Autodesk Fusion 360 part; units mm, degrees
(part 12 of 40)
  spline S70 degree 5 poles (151.3635, 144.3049) (151.3327, 144.3021) (151.2711, 144.2971) (151.1787, 144.2922) (151.0554, 144.2903) (150.901, 144.2944) (150.7464, 144.3031) (150.5917, 144.3146) (150.437, 144.3277) (150.2822, 144.3417) (150.1275, 144.3569) (149.9727, 144.3735) (149.818, 144.392) (149.6632, 144.4129) (149.5085, 144.4359) (149.3538, 144.461) (149.1991, 144.4879) (149.0445, 144.5162) (148.8899, 144.5458) (148.7354, 144.5767) (148.5809, 144.6087) (148.4265, 144.6421) (148.2722, 144.6768) (148.118, 144.7129) (147.9638, 144.7503) (147.8098, 144.7891) (147.6558, 144.8291) (147.5019, 144.8703) (147.3481, 144.9127) (147.1944, 144.9561) (147.0408, 145.0007) (146.8873, 145.0464) (146.734, 145.0932) (146.5807, 145.1411) (146.4276, 145.1901) (146.2746, 145.2401) (146.1217, 145.2913) (145.9689, 145.3434) (145.8162, 145.3965) (145.6637, 145.4507) (145.5114, 145.5058) (145.3591, 145.562) (145.207, 145.619) (145.055, 145.6771) (144.9032, 145.7361) (144.7516, 145.7961) (144.6, 145.857) (144.4487, 145.9188) (144.2975, 145.9815) (144.1464, 146.0452) (143.9955, 146.1097) (143.8448, 146.1751) (143.6942, 146.2415) (143.5438, 146.3087) (143.3936, 146.3767) (143.2435, 146.4457) (143.0936, 146.5154) (142.9439, 146.5861) (142.7944, 146.6575) (142.645, 146.7299) (142.4958, 146.803) (142.3468, 146.877) (142.198, 146.9518) (142.0494, 147.0274) (141.9009, 147.1038) (141.7527, 147.181) (141.6046, 147.259) (141.4568, 147.3378) (141.3091, 147.4174) (141.1617, 147.4977) (141.0144, 147.5789) (140.8968, 147.6444) (140.8086, 147.6939) (140.7499, 147.7271) (140.7205, 147.7437) knots 0 0 0 0 0 0 0.01428571 0.02857143 0.04285714 0.05714286 0.07142857 0.08571429 0.1 0.11428571 0.12857143 0.14285714 0.15714286 0.17142857 0.18571429 0.2 0.21428571 0.22857143 0.24285714 0.25714286 0.27142857 0.28571429 0.3 0.31428571 0.32857143 0.34285714 0.35714286 0.37142857 0.38571429 0.4 0.41428571 0.42857143 0.44285714 0.45714286 0.47142857 0.48571429 0.5 0.51428571 0.52857143 0.54285714 0.55714286 0.57142857 0.58571429 0.6 0.61428571 0.62857143 0.64285714 0.65714286 0.67142857 0.68571429 0.7 0.71428571 0.72857143 0.74285714 0.75714286 0.77142857 0.78571429 0.8 0.81428571 0.82857143 0.84285714 0.85714286 0.87142857 0.88571429 0.9 0.91428571 0.92857143 0.94285714 0.95714286 0.97142857 0.98571429 1 1 1 1 1 1
  line L5257 (151.3635, 144.3049) -> (151.3327, 144.3021) construction
  line L5258 (151.3327, 144.3021) -> (151.2711, 144.2971) construction
  line L5259 (151.2711, 144.2971) -> (151.1787, 144.2922) construction
  line L5260 (151.1787, 144.2922) -> (151.0554, 144.2903) construction
  line L5261 (151.0554, 144.2903) -> (150.901, 144.2944) construction
  line L5262 (150.901, 144.2944) -> (150.7464, 144.3031) construction
  line L5263 (150.7464, 144.3031) -> (150.5917, 144.3146) construction
  line L5264 (150.5917, 144.3146) -> (150.437, 144.3277) construction
  line L5265 (150.437, 144.3277) -> (150.2822, 144.3417) construction
  line L5266 (150.2822, 144.3417) -> (150.1275, 144.3569) construction
  line L5267 (150.1275, 144.3569) -> (149.9727, 144.3735) construction
  line L5268 (149.9727, 144.3735) -> (149.818, 144.392) construction
  line L5269 (149.818, 144.392) -> (149.6632, 144.4129) construction
  line L5270 (149.6632, 144.4129) -> (149.5085, 144.4359) construction
  line L5271 (149.5085, 144.4359) -> (149.3538, 144.461) construction
  line L5272 (149.3538, 144.461) -> (149.1991, 144.4879) construction
  line L5273 (149.1991, 144.4879) -> (149.0445, 144.5162) construction
  line L5274 (149.0445, 144.5162) -> (148.8899, 144.5458) construction
  line L5275 (148.8899, 144.5458) -> (148.7354, 144.5767) construction
  line L5276 (148.7354, 144.5767) -> (148.5809, 144.6087) construction
  line L5277 (148.5809, 144.6087) -> (148.4265, 144.6421) construction
  line L5278 (148.4265, 144.6421) -> (148.2722, 144.6768) construction
  line L5279 (148.2722, 144.6768) -> (148.118, 144.7129) construction
  line L5280 (148.118, 144.7129) -> (147.9638, 144.7503) construction
  line L5281 (147.9638, 144.7503) -> (147.8098, 144.7891) construction
  line L5282 (147.8098, 144.7891) -> (147.6558, 144.8291) construction
  line L5283 (147.6558, 144.8291) -> (147.5019, 144.8703) construction
  line L5284 (147.5019, 144.8703) -> (147.3481, 144.9127) construction
  line L5285 (147.3481, 144.9127) -> (147.1944, 144.9561) construction
  line L5286 (147.1944, 144.9561) -> (147.0408, 145.0007) construction
  line L5287 (147.0408, 145.0007) -> (146.8873, 145.0464) construction
  line L5288 (146.8873, 145.0464) -> (146.734, 145.0932) construction
  line L5289 (146.734, 145.0932) -> (146.5807, 145.1411) construction
  line L5290 (146.5807, 145.1411) -> (146.4276, 145.1901) construction
  line L5291 (146.4276, 145.1901) -> (146.2746, 145.2401) construction
  line L5292 (146.2746, 145.2401) -> (146.1217, 145.2913) construction
  line L5293 (146.1217, 145.2913) -> (145.9689, 145.3434) construction
  line L5294 (145.9689, 145.3434) -> (145.8162, 145.3965) construction
  line L5295 (145.8162, 145.3965) -> (145.6637, 145.4507) construction
  line L5296 (145.6637, 145.4507) -> (145.5114, 145.5058) construction
  line L5297 (145.5114, 145.5058) -> (145.3591, 145.562) construction
  line L5298 (145.3591, 145.562) -> (145.207, 145.619) construction
  line L5299 (145.207, 145.619) -> (145.055, 145.6771) construction
  line L5300 (145.055, 145.6771) -> (144.9032, 145.7361) construction
  line L5301 (144.9032, 145.7361) -> (144.7516, 145.7961) construction
  line L5302 (144.7516, 145.7961) -> (144.6, 145.857) construction
  line L5303 (144.6, 145.857) -> (144.4487, 145.9188) construction
  line L5304 (144.4487, 145.9188) -> (144.2975, 145.9815) construction
  line L5305 (144.2975, 145.9815) -> (144.1464, 146.0452) construction
  line L5306 (144.1464, 146.0452) -> (143.9955, 146.1097) construction
  line L5307 (143.9955, 146.1097) -> (143.8448, 146.1751) construction
  line L5308 (143.8448, 146.1751) -> (143.6942, 146.2415) construction
  line L5309 (143.6942, 146.2415) -> (143.5438, 146.3087) construction
  line L5310 (143.5438, 146.3087) -> (143.3936, 146.3767) construction
  line L5311 (143.3936, 146.3767) -> (143.2435, 146.4457) construction
  line L5312 (143.2435, 146.4457) -> (143.0936, 146.5154) construction
  line L5313 (143.0936, 146.5154) -> (142.9439, 146.5861) construction
  line L5314 (142.9439, 146.5861) -> (142.7944, 146.6575) construction
  line L5315 (142.7944, 146.6575) -> (142.645, 146.7299) construction
  line L5316 (142.645, 146.7299) -> (142.4958, 146.803) construction
  line L5317 (142.4958, 146.803) -> (142.3468, 146.877) construction
  line L5318 (142.3468, 146.877) -> (142.198, 146.9518) construction
  line L5319 (142.198, 146.9518) -> (142.0494, 147.0274) construction
  line L5320 (142.0494, 147.0274) -> (141.9009, 147.1038) construction
  line L5321 (141.9009, 147.1038) -> (141.7527, 147.181) construction
  line L5322 (141.7527, 147.181) -> (141.6046, 147.259) construction
  line L5323 (141.6046, 147.259) -> (141.4568, 147.3378) construction
  line L5324 (141.4568, 147.3378) -> (141.3091, 147.4174) construction
  line L5325 (141.3091, 147.4174) -> (141.1617, 147.4977) construction
  line L5326 (141.1617, 147.4977) -> (141.0144, 147.5789) construction
  line L5327 (141.0144, 147.5789) -> (140.8968, 147.6444) construction
  line L5328 (140.8968, 147.6444) -> (140.8086, 147.6939) construction
  line L5329 (140.8086, 147.6939) -> (140.7499, 147.7271) construction
  line L5330 (140.7499, 147.7271) -> (140.7205, 147.7437) construction
  arc A144 (140.7205, 152.2563) -> (140.7205, 147.7437) centre (212.132, 150) ccw
  spline S71 degree 5 poles (159.6217, 118.8885) (159.5952, 118.8728) (159.5425, 118.8406) (159.4648, 118.7903) (159.3639, 118.7193) (159.2414, 118.6252) (159.1214, 118.5273) (159.0031, 118.4271) (158.8856, 118.3256) (158.7686, 118.2233) (158.6523, 118.12) (158.5369, 118.0156) (158.4226, 117.9097) (158.3096, 117.8019) (158.198, 117.6923) (158.0876, 117.581) (157.9783, 117.4684) (157.8698, 117.3545) (157.7622, 117.2397) (157.6553, 117.124) (157.5492, 117.0073) (157.4439, 116.8895) (157.3394, 116.7708) (157.2359, 116.6509) (157.1332, 116.53) (157.0313, 116.4081) (156.9303, 116.2852) (156.83, 116.1614) (156.7305, 116.0367) (156.6317, 115.9112) (156.5336, 115.7849) (156.4363, 115.6577) (156.3397, 115.5297) (156.2439, 115.4009) (156.1488, 115.2712) (156.0544, 115.1408) (155.9608, 115.0095) (155.8678, 114.8776) (155.7756, 114.7448) (155.684, 114.6114) (155.5932, 114.4772) (155.503, 114.3423) (155.4135, 114.2067) (155.3247, 114.0705) (155.2365, 113.9335) (155.1491, 113.7958) (155.0623, 113.6575) (154.9762, 113.5185) (154.8907, 113.3789) (154.8059, 113.2386) (154.7218, 113.0977) (154.6383, 112.9562) (154.5555, 112.814) (154.4733, 112.6712) (154.3917, 112.5279) (154.3108, 112.3839) (154.2306, 112.2393) (154.151, 112.0942) (154.072, 111.9485) (153.9937, 111.8022) (153.916, 111.6553) (153.8389, 111.5079) (153.7625, 111.3599) (153.6867, 111.2114) (153.6115, 111.0623) (153.537, 110.9127) (153.463, 110.7626) (153.3897, 110.6119) (153.3171, 110.4607) (153.245, 110.3091) (153.1736, 110.1569) (153.1169, 110.0347) (153.0747, 109.9428) (153.0467, 109.8815) (153.0327, 109.8508) knots 0 0 0 0 0 0 0.01428571 0.02857143 0.04285714 0.05714286 0.07142857 0.08571429 0.1 0.11428571 0.12857143 0.14285714 0.15714286 0.17142857 0.18571429 0.2 0.21428571 0.22857143 0.24285714 0.25714286 0.27142857 0.28571429 0.3 0.31428571 0.32857143 0.34285714 0.35714286 0.37142857 0.38571429 0.4 0.41428571 0.42857143 0.44285714 0.45714286 0.47142857 0.48571429 0.5 0.51428571 0.52857143 0.54285714 0.55714286 0.57142857 0.58571429 0.6 0.61428571 0.62857143 0.64285714 0.65714286 0.67142857 0.68571429 0.7 0.71428571 0.72857143 0.74285714 0.75714286 0.77142857 0.78571429 0.8 0.81428571 0.82857143 0.84285714 0.85714286 0.87142857 0.88571429 0.9 0.91428571 0.92857143 0.94285714 0.95714286 0.97142857 0.98571429 1 1 1 1 1 1
  line L5331 (159.6217, 118.8885) -> (159.5952, 118.8728) construction
  line L5332 (159.5952, 118.8728) -> (159.5425, 118.8406) construction
  line L5333 (159.5425, 118.8406) -> (159.4648, 118.7903) construction
  line L5334 (159.4648, 118.7903) -> (159.3639, 118.7193) construction
  line L5335 (159.3639, 118.7193) -> (159.2414, 118.6252) construction
  line L5336 (159.2414, 118.6252) -> (159.1214, 118.5273) construction
  line L5337 (159.1214, 118.5273) -> (159.0031, 118.4271) construction
  line L5338 (159.0031, 118.4271) -> (158.8856, 118.3256) construction
  line L5339 (158.8856, 118.3256) -> (158.7686, 118.2233) construction
  line L5340 (158.7686, 118.2233) -> (158.6523, 118.12) construction
  line L5341 (158.6523, 118.12) -> (158.5369, 118.0156) construction
  line L5342 (158.5369, 118.0156) -> (158.4226, 117.9097) construction
  line L5343 (158.4226, 117.9097) -> (158.3096, 117.8019) construction
  line L5344 (158.3096, 117.8019) -> (158.198, 117.6923) construction
  line L5345 (158.198, 117.6923) -> (158.0876, 117.581) construction
  line L5346 (158.0876, 117.581) -> (157.9783, 117.4684) construction
  line L5347 (157.9783, 117.4684) -> (157.8698, 117.3545) construction
  line L5348 (157.8698, 117.3545) -> (157.7622, 117.2397) construction
  line L5349 (157.7622, 117.2397) -> (157.6553, 117.124) construction
  line L5350 (157.6553, 117.124) -> (157.5492, 117.0073) construction
  line L5351 (157.5492, 117.0073) -> (157.4439, 116.8895) construction
  line L5352 (157.4439, 116.8895) -> (157.3394, 116.7708) construction
  line L5353 (157.3394, 116.7708) -> (157.2359, 116.6509) construction
  line L5354 (157.2359, 116.6509) -> (157.1332, 116.53) construction
  line L5355 (157.1332, 116.53) -> (157.0313, 116.4081) construction
  line L5356 (157.0313, 116.4081) -> (156.9303, 116.2852) construction
  line L5357 (156.9303, 116.2852) -> (156.83, 116.1614) construction
  line L5358 (156.83, 116.1614) -> (156.7305, 116.0367) construction
  line L5359 (156.7305, 116.0367) -> (156.6317, 115.9112) construction
  line L5360 (156.6317, 115.9112) -> (156.5336, 115.7849) construction
  line L5361 (156.5336, 115.7849) -> (156.4363, 115.6577) construction
  line L5362 (156.4363, 115.6577) -> (156.3397, 115.5297) construction
  line L5363 (156.3397, 115.5297) -> (156.2439, 115.4009) construction
  line L5364 (156.2439, 115.4009) -> (156.1488, 115.2712) construction
  line L5365 (156.1488, 115.2712) -> (156.0544, 115.1408) construction
  line L5366 (156.0544, 115.1408) -> (155.9608, 115.0095) construction
  line L5367 (155.9608, 115.0095) -> (155.8678, 114.8776) construction
  line L5368 (155.8678, 114.8776) -> (155.7756, 114.7448) construction
  line L5369 (155.7756, 114.7448) -> (155.684, 114.6114) construction
  line L5370 (155.684, 114.6114) -> (155.5932, 114.4772) construction
  line L5371 (155.5932, 114.4772) -> (155.503, 114.3423) construction
  line L5372 (155.503, 114.3423) -> (155.4135, 114.2067) construction
  line L5373 (155.4135, 114.2067) -> (155.3247, 114.0705) construction
  line L5374 (155.3247, 114.0705) -> (155.2365, 113.9335) construction
  line L5375 (155.2365, 113.9335) -> (155.1491, 113.7958) construction
  line L5376 (155.1491, 113.7958) -> (155.0623, 113.6575) construction
  line L5377 (155.0623, 113.6575) -> (154.9762, 113.5185) construction
  line L5378 (154.9762, 113.5185) -> (154.8907, 113.3789) construction
  line L5379 (154.8907, 113.3789) -> (154.8059, 113.2386) construction
  line L5380 (154.8059, 113.2386) -> (154.7218, 113.0977) construction
  line L5381 (154.7218, 113.0977) -> (154.6383, 112.9562) construction
  line L5382 (154.6383, 112.9562) -> (154.5555, 112.814) construction
  line L5383 (154.5555, 112.814) -> (154.4733, 112.6712) construction
  line L5384 (154.4733, 112.6712) -> (154.3917, 112.5279) construction
  line L5385 (154.3917, 112.5279) -> (154.3108, 112.3839) construction
  line L5386 (154.3108, 112.3839) -> (154.2306, 112.2393) construction
  line L5387 (154.2306, 112.2393) -> (154.151, 112.0942) construction
  line L5388 (154.151, 112.0942) -> (154.072, 111.9485) construction
  line L5389 (154.072, 111.9485) -> (153.9937, 111.8022) construction
  line L5390 (153.9937, 111.8022) -> (153.916, 111.6553) construction
  line L5391 (153.916, 111.6553) -> (153.8389, 111.5079) construction
  line L5392 (153.8389, 111.5079) -> (153.7625, 111.3599) construction
  line L5393 (153.7625, 111.3599) -> (153.6867, 111.2114) construction
  line L5394 (153.6867, 111.2114) -> (153.6115, 111.0623) construction
  line L5395 (153.6115, 111.0623) -> (153.537, 110.9127) construction
  line L5396 (153.537, 110.9127) -> (153.463, 110.7626) construction
  line L5397 (153.463, 110.7626) -> (153.3897, 110.6119) construction
  line L5398 (153.3897, 110.6119) -> (153.3171, 110.4607) construction
  line L5399 (153.3171, 110.4607) -> (153.245, 110.3091) construction
  line L5400 (153.245, 110.3091) -> (153.1736, 110.1569) construction
  line L5401 (153.1736, 110.1569) -> (153.1169, 110.0347) construction
  line L5402 (153.1169, 110.0347) -> (153.0747, 109.9428) construction
  line L5403 (153.0747, 109.9428) -> (153.0467, 109.8815) construction
  line L5404 (153.0467, 109.8815) -> (153.0327, 109.8508) construction
  arc A145 (152.9878, 155.5428) -> (155.1583, 157.2806) centre (153.1745, 157.5341) ccw
  arc A146 (160.1966, 125.4699) -> (157.5954, 126.4519) centre (158.3882, 124.6158) ccw
  arc A147 (155.6851, 193.8) -> (153.0327, 190.1492) centre (212.132, 150) ccw
  spline S72 degree 5 poles (152.5778, 136.6378) (152.5477, 136.631) (152.4876, 136.6167) (152.3982, 136.5929) (152.2803, 136.5565) (152.1347, 136.5049) (151.9904, 136.4489) (151.8468, 136.3901) (151.7037, 136.3299) (151.5609, 136.2687) (151.4184, 136.2065) (151.2763, 136.1429) (151.1349, 136.0774) (150.9941, 136.0098) (150.8541, 135.94) (150.7147, 135.8684) (150.5759, 135.795) (150.4376, 135.7203) (150.2998, 135.6443) (150.1623, 135.5673) (150.0253, 135.4891) (149.8888, 135.4096) (149.7528, 135.3289) (149.6172, 135.247) (149.4822, 135.1637) (149.3477, 135.0792) (149.2136, 134.9936) (149.08, 134.9068) (148.9468, 134.819) (148.814, 134.7302) (148.6817, 134.6403) (148.5499, 134.5494) (148.4185, 134.4575) (148.2875, 134.3646) (148.157, 134.2707) (148.027, 134.1758) (147.8974, 134.08) (147.7682, 133.9832) (147.6394, 133.8854) (147.5111, 133.7868) (147.3832, 133.6873) (147.2558, 133.5869) (147.1288, 133.4856) (147.0022, 133.3834) (146.876, 133.2804) (146.7503, 133.1765) (146.625, 133.0717) (146.5002, 132.9662) (146.3758, 132.8598) (146.2518, 132.7526) (146.1282, 132.6445) (146.0051, 132.5357) (145.8823, 132.4261) (145.7601, 132.3158) (145.6382, 132.2046) (145.5168, 132.0927) (145.3958, 131.98) (145.2752, 131.8665) (145.1551, 131.7523) (145.0354, 131.6374) (144.9161, 131.5218) (144.7973, 131.4054) (144.6789, 131.2882) (144.5609, 131.1704) (144.4433, 131.0519) (144.3262, 130.9326) (144.2095, 130.8127) (144.0932, 130.6921) (143.9774, 130.5707) (143.862, 130.4488) (143.747, 130.3261) (143.6553, 130.2274) (143.5868, 130.1531) (143.5412, 130.1034) (143.5184, 130.0785) knots 0 0 0 0 0 0 0.01428571 0.02857143 0.04285714 0.05714286 0.07142857 0.08571429 0.1 0.11428571 0.12857143 0.14285714 0.15714286 0.17142857 0.18571429 0.2 0.21428571 0.22857143 0.24285714 0.25714286 0.27142857 0.28571429 0.3 0.31428571 0.32857143 0.34285714 0.35714286 0.37142857 0.38571429 0.4 0.41428571 0.42857143 0.44285714 0.45714286 0.47142857 0.48571429 0.5 0.51428571 0.52857143 0.54285714 0.55714286 0.57142857 0.58571429 0.6 0.61428571 0.62857143 0.64285714 0.65714286 0.67142857 0.68571429 0.7 0.71428571 0.72857143 0.74285714 0.75714286 0.77142857 0.78571429 0.8 0.81428571 0.82857143 0.84285714 0.85714286 0.87142857 0.88571429 0.9 0.91428571 0.92857143 0.94285714 0.95714286 0.97142857 0.98571429 1 1 1 1 1 1
  line L5405 (152.5778, 136.6378) -> (152.5477, 136.631) construction
  line L5406 (152.5477, 136.631) -> (152.4876, 136.6167) construction
  line L5407 (152.4876, 136.6167) -> (152.3982, 136.5929) construction
  line L5408 (152.3982, 136.5929) -> (152.2803, 136.5565) construction
  line L5409 (152.2803, 136.5565) -> (152.1347, 136.5049) construction
  line L5410 (152.1347, 136.5049) -> (151.9904, 136.4489) construction
  line L5411 (151.9904, 136.4489) -> (151.8468, 136.3901) construction
  line L5412 (151.8468, 136.3901) -> (151.7037, 136.3299) construction
  line L5413 (151.7037, 136.3299) -> (151.5609, 136.2687) construction
  line L5414 (151.5609, 136.2687) -> (151.4184, 136.2065) construction
  line L5415 (151.4184, 136.2065) -> (151.2763, 136.1429) construction
  line L5416 (151.2763, 136.1429) -> (151.1349, 136.0774) construction
  line L5417 (151.1349, 136.0774) -> (150.9941, 136.0098) construction
  line L5418 (150.9941, 136.0098) -> (150.8541, 135.94) construction
  line L5419 (150.8541, 135.94) -> (150.7147, 135.8684) construction
  line L5420 (150.7147, 135.8684) -> (150.5759, 135.795) construction
  line L5421 (150.5759, 135.795) -> (150.4376, 135.7203) construction
  line L5422 (150.4376, 135.7203) -> (150.2998, 135.6443) construction
  line L5423 (150.2998, 135.6443) -> (150.1623, 135.5673) construction
  line L5424 (150.1623, 135.5673) -> (150.0253, 135.4891) construction
  line L5425 (150.0253, 135.4891) -> (149.8888, 135.4096) construction
  line L5426 (149.8888, 135.4096) -> (149.7528, 135.3289) construction
  line L5427 (149.7528, 135.3289) -> (149.6172, 135.247) construction
  line L5428 (149.6172, 135.247) -> (149.4822, 135.1637) construction
  line L5429 (149.4822, 135.1637) -> (149.3477, 135.0792) construction
  line L5430 (149.3477, 135.0792) -> (149.2136, 134.9936) construction
  line L5431 (149.2136, 134.9936) -> (149.08, 134.9068) construction
  line L5432 (149.08, 134.9068) -> (148.9468, 134.819) construction
  line L5433 (148.9468, 134.819) -> (148.814, 134.7302) construction
  line L5434 (148.814, 134.7302) -> (148.6817, 134.6403) construction
  line L5435 (148.6817, 134.6403) -> (148.5499, 134.5494) construction
  line L5436 (148.5499, 134.5494) -> (148.4185, 134.4575) construction
  line L5437 (148.4185, 134.4575) -> (148.2875, 134.3646) construction
  line L5438 (148.2875, 134.3646) -> (148.157, 134.2707) construction
  line L5439 (148.157, 134.2707) -> (148.027, 134.1758) construction
  line L5440 (148.027, 134.1758) -> (147.8974, 134.08) construction
  line L5441 (147.8974, 134.08) -> (147.7682, 133.9832) construction
  line L5442 (147.7682, 133.9832) -> (147.6394, 133.8854) construction
  line L5443 (147.6394, 133.8854) -> (147.5111, 133.7868) construction
  line L5444 (147.5111, 133.7868) -> (147.3832, 133.6873) construction
  line L5445 (147.3832, 133.6873) -> (147.2558, 133.5869) construction
  line L5446 (147.2558, 133.5869) -> (147.1288, 133.4856) construction
  line L5447 (147.1288, 133.4856) -> (147.0022, 133.3834) construction
  line L5448 (147.0022, 133.3834) -> (146.876, 133.2804) construction
  line L5449 (146.876, 133.2804) -> (146.7503, 133.1765) construction
  line L5450 (146.7503, 133.1765) -> (146.625, 133.0717) construction
  line L5451 (146.625, 133.0717) -> (146.5002, 132.9662) construction
  line L5452 (146.5002, 132.9662) -> (146.3758, 132.8598) construction
  line L5453 (146.3758, 132.8598) -> (146.2518, 132.7526) construction
  line L5454 (146.2518, 132.7526) -> (146.1282, 132.6445) construction
  line L5455 (146.1282, 132.6445) -> (146.0051, 132.5357) construction
  line L5456 (146.0051, 132.5357) -> (145.8823, 132.4261) construction
  line L5457 (145.8823, 132.4261) -> (145.7601, 132.3158) construction
  line L5458 (145.7601, 132.3158) -> (145.6382, 132.2046) construction
  line L5459 (145.6382, 132.2046) -> (145.5168, 132.0927) construction
  line L5460 (145.5168, 132.0927) -> (145.3958, 131.98) construction
  line L5461 (145.3958, 131.98) -> (145.2752, 131.8665) construction
  line L5462 (145.2752, 131.8665) -> (145.1551, 131.7523) construction
  line L5463 (145.1551, 131.7523) -> (145.0354, 131.6374) construction
  line L5464 (145.0354, 131.6374) -> (144.9161, 131.5218) construction
  line L5465 (144.9161, 131.5218) -> (144.7973, 131.4054) construction
  line L5466 (144.7973, 131.4054) -> (144.6789, 131.2882) construction
  line L5467 (144.6789, 131.2882) -> (144.5609, 131.1704) construction
  line L5468 (144.5609, 131.1704) -> (144.4433, 131.0519) construction
  line L5469 (144.4433, 131.0519) -> (144.3262, 130.9326) construction
  line L5470 (144.3262, 130.9326) -> (144.2095, 130.8127) construction
  line L5471 (144.2095, 130.8127) -> (144.0932, 130.6921) construction
  line L5472 (144.0932, 130.6921) -> (143.9774, 130.5707) construction
  line L5473 (143.9774, 130.5707) -> (143.862, 130.4488) construction
  line L5474 (143.862, 130.4488) -> (143.747, 130.3261) construction
  line L5475 (143.747, 130.3261) -> (143.6553, 130.2274) construction
  line L5476 (143.6553, 130.2274) -> (143.5868, 130.1531) construction
  line L5477 (143.5868, 130.1531) -> (143.5412, 130.1034) construction
  line L5478 (143.5412, 130.1034) -> (143.5184, 130.0785) construction
  spline S73 degree 5 poles (151.3635, 155.6951) (151.3327, 155.6979) (151.2711, 155.7029) (151.1787, 155.7078) (151.0554, 155.7097) (150.901, 155.7056) (150.7464, 155.6969) (150.5917, 155.6854) (150.437, 155.6723) (150.2822, 155.6583) (150.1275, 155.6431) (149.9727, 155.6265) (149.818, 155.608) (149.6632, 155.5871) (149.5085, 155.5641) (149.3538, 155.539) (149.1991, 155.5121) (149.0445, 155.4838) (148.8899, 155.4542) (148.7354, 155.4233) (148.5809, 155.3913) (148.4265, 155.3579) (148.2722, 155.3232) (148.118, 155.2871) (147.9638, 155.2497) (147.8098, 155.2109) (147.6558, 155.1709) (147.5019, 155.1297) (147.3481, 155.0873) (147.1944, 155.0439) (147.0408, 154.9993) (146.8873, 154.9536) (146.734, 154.9068) (146.5807, 154.8589) (146.4276, 154.8099) (146.2746, 154.7599) (146.1217, 154.7087) (145.9689, 154.6566) (145.8162, 154.6035) (145.6637, 154.5493) (145.5114, 154.4942) (145.3591, 154.438) (145.207, 154.381) (145.055, 154.3229) (144.9032, 154.2639) (144.7516, 154.2039) (144.6, 154.143) (144.4487, 154.0812) (144.2975, 154.0185) (144.1464, 153.9548) (143.9955, 153.8903) (143.8448, 153.8249) (143.6942, 153.7585) (143.5438, 153.6913) (143.3936, 153.6233) (143.2435, 153.5543) (143.0936, 153.4846) (142.9439, 153.4139) (142.7944, 153.3425) (142.645, 153.2701) (142.4958, 153.197) (142.3468, 153.123) (142.198, 153.0482) (142.0494, 152.9726) (141.9009, 152.8962) (141.7527, 152.819) (141.6046, 152.741) (141.4568, 152.6622) (141.3091, 152.5826) (141.1617, 152.5023) (141.0144, 152.4211) (140.8968, 152.3556) (140.8086, 152.3061) (140.7499, 152.2729) (140.7205, 152.2563) knots 0 0 0 0 0 0 0.01428571 0.02857143 0.04285714 0.05714286 0.07142857 0.08571429 0.1 0.11428571 0.12857143 0.14285714 0.15714286 0.17142857 0.18571429 0.2 0.21428571 0.22857143 0.24285714 0.25714286 0.27142857 0.28571429 0.3 0.31428571 0.32857143 0.34285714 0.35714286 0.37142857 0.38571429 0.4 0.41428571 0.42857143 0.44285714 0.45714286 0.47142857 0.48571429 0.5 0.51428571 0.52857143 0.54285714 0.55714286 0.57142857 0.58571429 0.6 0.61428571 0.62857143 0.64285714 0.65714286 0.67142857 0.68571429 0.7 0.71428571 0.72857143 0.74285714 0.75714286 0.77142857 0.78571429 0.8 0.81428571 0.82857143 0.84285714 0.85714286 0.87142857 0.88571429 0.9 0.91428571 0.92857143 0.94285714 0.95714286 0.97142857 0.98571429 1 1 1 1 1 1
  line L5479 (151.3635, 155.6951) -> (151.3327, 155.6979) construction
  line L5480 (151.3327, 155.6979) -> (151.2711, 155.7029) construction
  line L5481 (151.2711, 155.7029) -> (151.1787, 155.7078) construction
  line L5482 (151.1787, 155.7078) -> (151.0554, 155.7097) construction
  line L5483 (151.0554, 155.7097) -> (150.901, 155.7056) construction
  line L5484 (150.901, 155.7056) -> (150.7464, 155.6969) construction
  line L5485 (150.7464, 155.6969) -> (150.5917, 155.6854) construction
  line L5486 (150.5917, 155.6854) -> (150.437, 155.6723) construction
  line L5487 (150.437, 155.6723) -> (150.2822, 155.6583) construction
  line L5488 (150.2822, 155.6583) -> (150.1275, 155.6431) construction
  line L5489 (150.1275, 155.6431) -> (149.9727, 155.6265) construction
  line L5490 (149.9727, 155.6265) -> (149.818, 155.608) construction
  line L5491 (149.818, 155.608) -> (149.6632, 155.5871) construction
  line L5492 (149.6632, 155.5871) -> (149.5085, 155.5641) construction
  line L5493 (149.5085, 155.5641) -> (149.3538, 155.539) construction
  line L5494 (149.3538, 155.539) -> (149.1991, 155.5121) construction
  line L5495 (149.1991, 155.5121) -> (149.0445, 155.4838) construction
  line L5496 (149.0445, 155.4838) -> (148.8899, 155.4542) construction
  line L5497 (148.8899, 155.4542) -> (148.7354, 155.4233) construction
  line L5498 (148.7354, 155.4233) -> (148.5809, 155.3913) construction
  line L5499 (148.5809, 155.3913) -> (148.4265, 155.3579) construction
  line L5500 (148.4265, 155.3579) -> (148.2722, 155.3232) construction
  line L5501 (148.2722, 155.3232) -> (148.118, 155.2871) construction
  line L5502 (148.118, 155.2871) -> (147.9638, 155.2497) construction
  line L5503 (147.9638, 155.2497) -> (147.8098, 155.2109) construction
  line L5504 (147.8098, 155.2109) -> (147.6558, 155.1709) construction
  line L5505 (147.6558, 155.1709) -> (147.5019, 155.1297) construction
  line L5506 (147.5019, 155.1297) -> (147.3481, 155.0873) construction
  line L5507 (147.3481, 155.0873) -> (147.1944, 155.0439) construction
  line L5508 (147.1944, 155.0439) -> (147.0408, 154.9993) construction
  line L5509 (147.0408, 154.9993) -> (146.8873, 154.9536) construction
  line L5510 (146.8873, 154.9536) -> (146.734, 154.9068) construction
  line L5511 (146.734, 154.9068) -> (146.5807, 154.8589) construction
  line L5512 (146.5807, 154.8589) -> (146.4276, 154.8099) construction
  line L5513 (146.4276, 154.8099) -> (146.2746, 154.7599) construction
  line L5514 (146.2746, 154.7599) -> (146.1217, 154.7087) construction
  line L5515 (146.1217, 154.7087) -> (145.9689, 154.6566) construction
  line L5516 (145.9689, 154.6566) -> (145.8162, 154.6035) construction
  line L5517 (145.8162, 154.6035) -> (145.6637, 154.5493) construction
  line L5518 (145.6637, 154.5493) -> (145.5114, 154.4942) construction
  line L5519 (145.5114, 154.4942) -> (145.3591, 154.438) construction
  line L5520 (145.3591, 154.438) -> (145.207, 154.381) construction
  line L5521 (145.207, 154.381) -> (145.055, 154.3229) construction
  line L5522 (145.055, 154.3229) -> (144.9032, 154.2639) construction
  line L5523 (144.9032, 154.2639) -> (144.7516, 154.2039) construction
  line L5524 (144.7516, 154.2039) -> (144.6, 154.143) construction
  line L5525 (144.6, 154.143) -> (144.4487, 154.0812) construction
  line L5526 (144.4487, 154.0812) -> (144.2975, 154.0185) construction
  line L5527 (144.2975, 154.0185) -> (144.1464, 153.9548) construction
  line L5528 (144.1464, 153.9548) -> (143.9955, 153.8903) construction
  line L5529 (143.9955, 153.8903) -> (143.8448, 153.8249) construction
  line L5530 (143.8448, 153.8249) -> (143.6942, 153.7585) construction
  line L5531 (143.6942, 153.7585) -> (143.5438, 153.6913) construction
  line L5532 (143.5438, 153.6913) -> (143.3936, 153.6233) construction
  line L5533 (143.3936, 153.6233) -> (143.2435, 153.5543) construction
  line L5534 (143.2435, 153.5543) -> (143.0936, 153.4846) construction
  line L5535 (143.0936, 153.4846) -> (142.9439, 153.4139) construction
  line L5536 (142.9439, 153.4139) -> (142.7944, 153.3425) construction
  line L5537 (142.7944, 153.3425) -> (142.645, 153.2701) construction
  line L5538 (142.645, 153.2701) -> (142.4958, 153.197) construction
  line L5539 (142.4958, 153.197) -> (142.3468, 153.123) construction
  line L5540 (142.3468, 153.123) -> (142.198, 153.0482) construction
  line L5541 (142.198, 153.0482) -> (142.0494, 152.9726) construction
  line L5542 (142.0494, 152.9726) -> (141.9009, 152.8962) construction
  line L5543 (141.9009, 152.8962) -> (141.7527, 152.819) construction
  line L5544 (141.7527, 152.819) -> (141.6046, 152.741) construction
  line L5545 (141.6046, 152.741) -> (141.4568, 152.6622) construction
  line L5546 (141.4568, 152.6622) -> (141.3091, 152.5826) construction
  line L5547 (141.3091, 152.5826) -> (141.1617, 152.5023) construction
  line L5548 (141.1617, 152.5023) -> (141.0144, 152.4211) construction
  line L5549 (141.0144, 152.4211) -> (140.8968, 152.3556) construction
  line L5550 (140.8968, 152.3556) -> (140.8086, 152.3061) construction
  line L5551 (140.8086, 152.3061) -> (140.7499, 152.2729) construction
  line L5552 (140.7499, 152.2729) -> (140.7205, 152.2563) construction
  arc A148 (155.1583, 142.7194) -> (155.697, 139.3184) centre (212.132, 150) ccw
  spline S74 degree 5 poles (159.6217, 181.1115) (159.5952, 181.1272) (159.5425, 181.1594) (159.4648, 181.2097) (159.3639, 181.2807) (159.2414, 181.3748) (159.1214, 181.4727) (159.0031, 181.5729) (158.8856, 181.6744) (158.7686, 181.7767) (158.6523, 181.88) (158.5369, 181.9844) (158.4226, 182.0903) (158.3096, 182.1981) (158.198, 182.3077) (158.0876, 182.419) (157.9783, 182.5316) (157.8698, 182.6455) (157.7622, 182.7603) (157.6553, 182.876) (157.5492, 182.9927) (157.4439, 183.1105) (157.3394, 183.2292) (157.2359, 183.3491) (157.1332, 183.47) (157.0313, 183.5919) (156.9303, 183.7148) (156.83, 183.8386) (156.7305, 183.9633) (156.6317, 184.0888) (156.5336, 184.2151) (156.4363, 184.3423) (156.3397, 184.4703) (156.2439, 184.5991) (156.1488, 184.7288) (156.0544, 184.8592) (155.9608, 184.9905) (155.8678, 185.1224) (155.7756, 185.2552) (155.684, 185.3886) (155.5932, 185.5228) (155.503, 185.6577) (155.4135, 185.7933) (155.3247, 185.9295) (155.2365, 186.0665) (155.1491, 186.2042) (155.0623, 186.3425) (154.9762, 186.4815) (154.8907, 186.6211) (154.8059, 186.7614) (154.7218, 186.9023) (154.6383, 187.0438) (154.5555, 187.186) (154.4733, 187.3288) (154.3917, 187.4721) (154.3108, 187.6161) (154.2306, 187.7607) (154.151, 187.9058) (154.072, 188.0515) (153.9937, 188.1978) (153.916, 188.3447) (153.8389, 188.4921) (153.7625, 188.6401) (153.6867, 188.7886) (153.6115, 188.9377) (153.537, 189.0873) (153.463, 189.2374) (153.3897, 189.3881) (153.3171, 189.5393) (153.245, 189.6909) (153.1736, 189.8431) (153.1169, 189.9653) (153.0747, 190.0572) (153.0467, 190.1185) (153.0327, 190.1492) knots 0 0 0 0 0 0 0.01428571 0.02857143 0.04285714 0.05714286 0.07142857 0.08571429 0.1 0.11428571 0.12857143 0.14285714 0.15714286 0.17142857 0.18571429 0.2 0.21428571 0.22857143 0.24285714 0.25714286 0.27142857 0.28571429 0.3 0.31428571 0.32857143 0.34285714 0.35714286 0.37142857 0.38571429 0.4 0.41428571 0.42857143 0.44285714 0.45714286 0.47142857 0.48571429 0.5 0.51428571 0.52857143 0.54285714 0.55714286 0.57142857 0.58571429 0.6 0.61428571 0.62857143 0.64285714 0.65714286 0.67142857 0.68571429 0.7 0.71428571 0.72857143 0.74285714 0.75714286 0.77142857 0.78571429 0.8 0.81428571 0.82857143 0.84285714 0.85714286 0.87142857 0.88571429 0.9 0.91428571 0.92857143 0.94285714 0.95714286 0.97142857 0.98571429 1 1 1 1 1 1
  line L5553 (159.6217, 181.1115) -> (159.5952, 181.1272) construction
  line L5554 (159.5952, 181.1272) -> (159.5425, 181.1594) construction
  line L5555 (159.5425, 181.1594) -> (159.4648, 181.2097) construction
  line L5556 (159.4648, 181.2097) -> (159.3639, 181.2807) construction
  line L5557 (159.3639, 181.2807) -> (159.2414, 181.3748) construction
  line L5558 (159.2414, 181.3748) -> (159.1214, 181.4727) construction
  line L5559 (159.1214, 181.4727) -> (159.0031, 181.5729) construction
  line L5560 (159.0031, 181.5729) -> (158.8856, 181.6744) construction
  line L5561 (158.8856, 181.6744) -> (158.7686, 181.7767) construction
  line L5562 (158.7686, 181.7767) -> (158.6523, 181.88) construction
  line L5563 (158.6523, 181.88) -> (158.5369, 181.9844) construction
  line L5564 (158.5369, 181.9844) -> (158.4226, 182.0903) construction
  line L5565 (158.4226, 182.0903) -> (158.3096, 182.1981) construction
  line L5566 (158.3096, 182.1981) -> (158.198, 182.3077) construction
  line L5567 (158.198, 182.3077) -> (158.0876, 182.419) construction
  line L5568 (158.0876, 182.419) -> (157.9783, 182.5316) construction
  line L5569 (157.9783, 182.5316) -> (157.8698, 182.6455) construction
  line L5570 (157.8698, 182.6455) -> (157.7622, 182.7603) construction
  line L5571 (157.7622, 182.7603) -> (157.6553, 182.876) construction
  line L5572 (157.6553, 182.876) -> (157.5492, 182.9927) construction
  line L5573 (157.5492, 182.9927) -> (157.4439, 183.1105) construction
  line L5574 (157.4439, 183.1105) -> (157.3394, 183.2292) construction
  line L5575 (157.3394, 183.2292) -> (157.2359, 183.3491) construction
  line L5576 (157.2359, 183.3491) -> (157.1332, 183.47) construction
  line L5577 (157.1332, 183.47) -> (157.0313, 183.5919) construction
  line L5578 (157.0313, 183.5919) -> (156.9303, 183.7148) construction
  line L5579 (156.9303, 183.7148) -> (156.83, 183.8386) construction
  line L5580 (156.83, 183.8386) -> (156.7305, 183.9633) construction
  line L5581 (156.7305, 183.9633) -> (156.6317, 184.0888) construction
  line L5582 (156.6317, 184.0888) -> (156.5336, 184.2151) construction
  line L5583 (156.5336, 184.2151) -> (156.4363, 184.3423) construction
  line L5584 (156.4363, 184.3423) -> (156.3397, 184.4703) construction
  line L5585 (156.3397, 184.4703) -> (156.2439, 184.5991) construction
  line L5586 (156.2439, 184.5991) -> (156.1488, 184.7288) construction
  line L5587 (156.1488, 184.7288) -> (156.0544, 184.8592) construction
  line L5588 (156.0544, 184.8592) -> (155.9608, 184.9905) construction
  line L5589 (155.9608, 184.9905) -> (155.8678, 185.1224) construction
  line L5590 (155.8678, 185.1224) -> (155.7756, 185.2552) construction
  line L5591 (155.7756, 185.2552) -> (155.684, 185.3886) construction
  line L5592 (155.684, 185.3886) -> (155.5932, 185.5228) construction
  line L5593 (155.5932, 185.5228) -> (155.503, 185.6577) construction
  line L5594 (155.503, 185.6577) -> (155.4135, 185.7933) construction
  line L5595 (155.4135, 185.7933) -> (155.3247, 185.9295) construction
  line L5596 (155.3247, 185.9295) -> (155.2365, 186.0665) construction
  line L5597 (155.2365, 186.0665) -> (155.1491, 186.2042) construction
  line L5598 (155.1491, 186.2042) -> (155.0623, 186.3425) construction
  line L5599 (155.0623, 186.3425) -> (154.9762, 186.4815) construction
  line L5600 (154.9762, 186.4815) -> (154.8907, 186.6211) construction
  line L5601 (154.8907, 186.6211) -> (154.8059, 186.7614) construction
  line L5602 (154.8059, 186.7614) -> (154.7218, 186.9023) construction
  line L5603 (154.7218, 186.9023) -> (154.6383, 187.0438) construction
  line L5604 (154.6383, 187.0438) -> (154.5555, 187.186) construction
  line L5605 (154.5555, 187.186) -> (154.4733, 187.3288) construction
  line L5606 (154.4733, 187.3288) -> (154.3917, 187.4721) construction
  line L5607 (154.3917, 187.4721) -> (154.3108, 187.6161) construction
  line L5608 (154.3108, 187.6161) -> (154.2306, 187.7607) construction
  line L5609 (154.2306, 187.7607) -> (154.151, 187.9058) construction
  line L5610 (154.151, 187.9058) -> (154.072, 188.0515) construction
  line L5611 (154.072, 188.0515) -> (153.9937, 188.1978) construction
  line L5612 (153.9937, 188.1978) -> (153.916, 188.3447) construction
  line L5613 (153.916, 188.3447) -> (153.8389, 188.4921) construction
  line L5614 (153.8389, 188.4921) -> (153.7625, 188.6401) construction
  line L5615 (153.7625, 188.6401) -> (153.6867, 188.7886) construction
  line L5616 (153.6867, 188.7886) -> (153.6115, 188.9377) construction
  line L5617 (153.6115, 188.9377) -> (153.537, 189.0873) construction
  line L5618 (153.537, 189.0873) -> (153.463, 189.2374) construction
  line L5619 (153.463, 189.2374) -> (153.3897, 189.3881) construction
  line L5620 (153.3897, 189.3881) -> (153.3171, 189.5393) construction
  line L5621 (153.3171, 189.5393) -> (153.245, 189.6909) construction
  line L5622 (153.245, 189.6909) -> (153.1736, 189.8431) construction
  line L5623 (153.1736, 189.8431) -> (153.1169, 189.9653) construction
  line L5624 (153.1169, 189.9653) -> (153.0747, 190.0572) construction
  line L5625 (153.0747, 190.0572) -> (153.0467, 190.1185) construction
  line L5626 (153.0467, 190.1185) -> (153.0327, 190.1492) construction
  line L5627 (154.1697, 163.005) -> (152.5778, 163.3622)
  line L5628 (154.1697, 163.005) -> (152.5778, 163.3622)
  line L5629 (154.1697, 136.995) -> (152.5778, 136.6378)
  line L5630 (161.0254, 180.2798) -> (159.6217, 181.1115)
  line L5631 (154.1697, 136.995) -> (152.5778, 136.6378)
  spline S75 degree 5 poles (159.6217, 118.8885) (159.5952, 118.8728) (159.5425, 118.8406) (159.4648, 118.7903) (159.3639, 118.7193) (159.2414, 118.6252) (159.1214, 118.5273) (159.0031, 118.4271) (158.8856, 118.3256) (158.7686, 118.2233) (158.6523, 118.12) (158.5369, 118.0156) (158.4226, 117.9097) (158.3096, 117.8019) (158.198, 117.6923) (158.0876, 117.581) (157.9783, 117.4684) (157.8698, 117.3545) (157.7622, 117.2397) (157.6553, 117.124) (157.5492, 117.0073) (157.4439, 116.8895) (157.3394, 116.7708) (157.2359, 116.6509) (157.1332, 116.53) (157.0313, 116.4081) (156.9303, 116.2852) (156.83, 116.1614) (156.7305, 116.0367) (156.6317, 115.9112) (156.5336, 115.7849) (156.4363, 115.6577) (156.3397, 115.5297) (156.2439, 115.4009) (156.1488, 115.2712) (156.0544, 115.1408) (155.9608, 115.0095) (155.8678, 114.8776) (155.7756, 114.7448) (155.684, 114.6114) (155.5932, 114.4772) (155.503, 114.3423) (155.4135, 114.2067) (155.3247, 114.0705) (155.2365, 113.9335) (155.1491, 113.7958) (155.0623, 113.6575) (154.9762, 113.5185) (154.8907, 113.3789) (154.8059, 113.2386) (154.7218, 113.0977) (154.6383, 112.9562) (154.5555, 112.814) (154.4733, 112.6712) (154.3917, 112.5279) (154.3108, 112.3839) (154.2306, 112.2393) (154.151, 112.0942) (154.072, 111.9485) (153.9937, 111.8022) (153.916, 111.6553) (153.8389, 111.5079) (153.7625, 111.3599) (153.6867, 111.2114) (153.6115, 111.0623) (153.537, 110.9127) (153.463, 110.7626) (153.3897, 110.6119) (153.3171, 110.4607) (153.245, 110.3091) (153.1736, 110.1569) (153.1169, 110.0347) (153.0747, 109.9428) (153.0467, 109.8815) (153.0327, 109.8508) knots 0 0 0 0 0 0 0.01428571 0.02857143 0.04285714 0.05714286 0.07142857 0.08571429 0.1 0.11428571 0.12857143 0.14285714 0.15714286 0.17142857 0.18571429 0.2 0.21428571 0.22857143 0.24285714 0.25714286 0.27142857 0.28571429 0.3 0.31428571 0.32857143 0.34285714 0.35714286 0.37142857 0.38571429 0.4 0.41428571 0.42857143 0.44285714 0.45714286 0.47142857 0.48571429 0.5 0.51428571 0.52857143 0.54285714 0.55714286 0.57142857 0.58571429 0.6 0.61428571 0.62857143 0.64285714 0.65714286 0.67142857 0.68571429 0.7 0.71428571 0.72857143 0.74285714 0.75714286 0.77142857 0.78571429 0.8 0.81428571 0.82857143 0.84285714 0.85714286 0.87142857 0.88571429 0.9 0.91428571 0.92857143 0.94285714 0.95714286 0.97142857 0.98571429 1 1 1 1 1 1
  line L5632 (159.6217, 118.8885) -> (159.5952, 118.8728) construction
  line L5633 (159.5952, 118.8728) -> (159.5425, 118.8406) construction
  line L5634 (159.5425, 118.8406) -> (159.4648, 118.7903) construction
  line L5635 (159.4648, 118.7903) -> (159.3639, 118.7193) construction
  line L5636 (159.3639, 118.7193) -> (159.2414, 118.6252) construction
  line L5637 (159.2414, 118.6252) -> (159.1214, 118.5273) construction
  line L5638 (159.1214, 118.5273) -> (159.0031, 118.4271) construction
  line L5639 (159.0031, 118.4271) -> (158.8856, 118.3256) construction
  line L5640 (158.8856, 118.3256) -> (158.7686, 118.2233) construction
  line L5641 (158.7686, 118.2233) -> (158.6523, 118.12) construction
  line L5642 (158.6523, 118.12) -> (158.5369, 118.0156) construction
  line L5643 (158.5369, 118.0156) -> (158.4226, 117.9097) construction
  line L5644 (158.4226, 117.9097) -> (158.3096, 117.8019) construction
  line L5645 (158.3096, 117.8019) -> (158.198, 117.6923) construction
  line L5646 (158.198, 117.6923) -> (158.0876, 117.581) construction
  line L5647 (158.0876, 117.581) -> (157.9783, 117.4684) construction
  line L5648 (157.9783, 117.4684) -> (157.8698, 117.3545) construction
  line L5649 (157.8698, 117.3545) -> (157.7622, 117.2397) construction
  line L5650 (157.7622, 117.2397) -> (157.6553, 117.124) construction
  line L5651 (157.6553, 117.124) -> (157.5492, 117.0073) construction
  line L5652 (157.5492, 117.0073) -> (157.4439, 116.8895) construction
  line L5653 (157.4439, 116.8895) -> (157.3394, 116.7708) construction
  line L5654 (157.3394, 116.7708) -> (157.2359, 116.6509) construction
  line L5655 (157.2359, 116.6509) -> (157.1332, 116.53) construction
  line L5656 (157.1332, 116.53) -> (157.0313, 116.4081) construction
  line L5657 (157.0313, 116.4081) -> (156.9303, 116.2852) construction
  line L5658 (156.9303, 116.2852) -> (156.83, 116.1614) construction
  line L5659 (156.83, 116.1614) -> (156.7305, 116.0367) construction
  line L5660 (156.7305, 116.0367) -> (156.6317, 115.9112) construction
  line L5661 (156.6317, 115.9112) -> (156.5336, 115.7849) construction
  line L5662 (156.5336, 115.7849) -> (156.4363, 115.6577) construction
  line L5663 (156.4363, 115.6577) -> (156.3397, 115.5297) construction
  line L5664 (156.3397, 115.5297) -> (156.2439, 115.4009) construction
  line L5665 (156.2439, 115.4009) -> (156.1488, 115.2712) construction
  line L5666 (156.1488, 115.2712) -> (156.0544, 115.1408) construction
  line L5667 (156.0544, 115.1408) -> (155.9608, 115.0095) construction
  line L5668 (155.9608, 115.0095) -> (155.8678, 114.8776) construction
  line L5669 (155.8678, 114.8776) -> (155.7756, 114.7448) construction
  line L5670 (155.7756, 114.7448) -> (155.684, 114.6114) construction
  line L5671 (155.684, 114.6114) -> (155.5932, 114.4772) construction
  line L5672 (155.5932, 114.4772) -> (155.503, 114.3423) construction
  line L5673 (155.503, 114.3423) -> (155.4135, 114.2067) construction
  line L5674 (155.4135, 114.2067) -> (155.3247, 114.0705) construction
  line L5675 (155.3247, 114.0705) -> (155.2365, 113.9335) construction
  line L5676 (155.2365, 113.9335) -> (155.1491, 113.7958) construction
  line L5677 (155.1491, 113.7958) -> (155.0623, 113.6575) construction
  line L5678 (155.0623, 113.6575) -> (154.9762, 113.5185) construction
  line L5679 (154.9762, 113.5185) -> (154.8907, 113.3789) construction
  line L5680 (154.8907, 113.3789) -> (154.8059, 113.2386) construction
  line L5681 (154.8059, 113.2386) -> (154.7218, 113.0977) construction
  line L5682 (154.7218, 113.0977) -> (154.6383, 112.9562) construction
  line L5683 (154.6383, 112.9562) -> (154.5555, 112.814) construction
  line L5684 (154.5555, 112.814) -> (154.4733, 112.6712) construction
  line L5685 (154.4733, 112.6712) -> (154.3917, 112.5279) construction
  line L5686 (154.3917, 112.5279) -> (154.3108, 112.3839) construction
  line L5687 (154.3108, 112.3839) -> (154.2306, 112.2393) construction
  line L5688 (154.2306, 112.2393) -> (154.151, 112.0942) construction
  line L5689 (154.151, 112.0942) -> (154.072, 111.9485) construction
  line L5690 (154.072, 111.9485) -> (153.9937, 111.8022) construction
  line L5691 (153.9937, 111.8022) -> (153.916, 111.6553) construction
  line L5692 (153.916, 111.6553) -> (153.8389, 111.5079) construction
  line L5693 (153.8389, 111.5079) -> (153.7625, 111.3599) construction
  line L5694 (153.7625, 111.3599) -> (153.6867, 111.2114) construction
  line L5695 (153.6867, 111.2114) -> (153.6115, 111.0623) construction
  line L5696 (153.6115, 111.0623) -> (153.537, 110.9127) construction
  line L5697 (153.537, 110.9127) -> (153.463, 110.7626) construction
  line L5698 (153.463, 110.7626) -> (153.3897, 110.6119) construction
  line L5699 (153.3897, 110.6119) -> (153.3171, 110.4607) construction
  line L5700 (153.3171, 110.4607) -> (153.245, 110.3091) construction
  line L5701 (153.245, 110.3091) -> (153.1736, 110.1569) construction
  line L5702 (153.1736, 110.1569) -> (153.1169, 110.0347) construction
  line L5703 (153.1169, 110.0347) -> (153.0747, 109.9428) construction
  line L5704 (153.0747, 109.9428) -> (153.0467, 109.8815) construction
  line L5705 (153.0467, 109.8815) -> (153.0327, 109.8508) construction
  arc A149 (161.7599, 177.5982) -> (160.1966, 174.5301) centre (212.132, 150) ccw
  arc A150 (155.697, 160.6816) -> (155.1583, 157.2806) centre (212.132, 150) ccw
  arc A151 (155.1583, 142.7194) -> (152.9878, 144.4572) centre (153.1745, 142.4659) ccw
  arc A152 (160.1966, 125.4699) -> (161.7599, 122.4018) centre (212.132, 150) ccw
  line L5706 (152.9878, 144.4572) -> (151.3635, 144.3049)
  spline S76 degree 5 poles (152.5778, 136.6378) (152.5477, 136.631) (152.4876, 136.6167) (152.3982, 136.5929) (152.2803, 136.5565) (152.1347, 136.5049) (151.9904, 136.4489) (151.8468, 136.3901) (151.7037, 136.3299) (151.5609, 136.2687) (151.4184, 136.2065) (151.2763, 136.1429) (151.1349, 136.0774) (150.9941, 136.0098) (150.8541, 135.94) (150.7147, 135.8684) (150.5759, 135.795) (150.4376, 135.7203) (150.2998, 135.6443) (150.1623, 135.5673) (150.0253, 135.4891) (149.8888, 135.4096) (149.7528, 135.3289) (149.6172, 135.247) (149.4822, 135.1637) (149.3477, 135.0792) (149.2136, 134.9936) (149.08, 134.9068) (148.9468, 134.819) (148.814, 134.7302) (148.6817, 134.6403) (148.5499, 134.5494) (148.4185, 134.4575) (148.2875, 134.3646) (148.157, 134.2707) (148.027, 134.1758) (147.8974, 134.08) (147.7682, 133.9832) (147.6394, 133.8854) (147.5111, 133.7868) (147.3832, 133.6873) (147.2558, 133.5869) (147.1288, 133.4856) (147.0022, 133.3834) (146.876, 133.2804) (146.7503, 133.1765) (146.625, 133.0717) (146.5002, 132.9662) (146.3758, 132.8598) (146.2518, 132.7526) (146.1282, 132.6445) (146.0051, 132.5357) (145.8823, 132.4261) (145.7601, 132.3158) (145.6382, 132.2046) (145.5168, 132.0927) (145.3958, 131.98) (145.2752, 131.8665) (145.1551, 131.7523) (145.0354, 131.6374) (144.9161, 131.5218) (144.7973, 131.4054) (144.6789, 131.2882) (144.5609, 131.1704) (144.4433, 131.0519) (144.3262, 130.9326) (144.2095, 130.8127) (144.0932, 130.6921) (143.9774, 130.5707) (143.862, 130.4488) (143.747, 130.3261) (143.6553, 130.2274) (143.5868, 130.1531) (143.5412, 130.1034) (143.5184, 130.0785) knots 0 0 0 0 0 0 0.01428571 0.02857143 0.04285714 0.05714286 0.07142857 0.08571429 0.1 0.11428571 0.12857143 0.14285714 0.15714286 0.17142857 0.18571429 0.2 0.21428571 0.22857143 0.24285714 0.25714286 0.27142857 0.28571429 0.3 0.31428571 0.32857143 0.34285714 0.35714286 0.37142857 0.38571429 0.4 0.41428571 0.42857143 0.44285714 0.45714286 0.47142857 0.48571429 0.5 0.51428571 0.52857143 0.54285714 0.55714286 0.57142857 0.58571429 0.6 0.61428571 0.62857143 0.64285714 0.65714286 0.67142857 0.68571429 0.7 0.71428571 0.72857143 0.74285714 0.75714286 0.77142857 0.78571429 0.8 0.81428571 0.82857143 0.84285714 0.85714286 0.87142857 0.88571429 0.9 0.91428571 0.92857143 0.94285714 0.95714286 0.97142857 0.98571429 1 1 1 1 1 1
  line L5707 (152.5778, 136.6378) -> (152.5477, 136.631) construction
  line L5708 (152.5477, 136.631) -> (152.4876, 136.6167) construction
  line L5709 (152.4876, 136.6167) -> (152.3982, 136.5929) construction
  line L5710 (152.3982, 136.5929) -> (152.2803, 136.5565) construction
  line L5711 (152.2803, 136.5565) -> (152.1347, 136.5049) construction
  line L5712 (152.1347, 136.5049) -> (151.9904, 136.4489) construction
  line L5713 (151.9904, 136.4489) -> (151.8468, 136.3901) construction
  line L5714 (151.8468, 136.3901) -> (151.7037, 136.3299) construction
  line L5715 (151.7037, 136.3299) -> (151.5609, 136.2687) construction
  line L5716 (151.5609, 136.2687) -> (151.4184, 136.2065) construction
  line L5717 (151.4184, 136.2065) -> (151.2763, 136.1429) construction
  line L5718 (151.2763, 136.1429) -> (151.1349, 136.0774) construction
  line L5719 (151.1349, 136.0774) -> (150.9941, 136.0098) construction
  line L5720 (150.9941, 136.0098) -> (150.8541, 135.94) construction
  line L5721 (150.8541, 135.94) -> (150.7147, 135.8684) construction
  line L5722 (150.7147, 135.8684) -> (150.5759, 135.795) construction
  line L5723 (150.5759, 135.795) -> (150.4376, 135.7203) construction
  line L5724 (150.4376, 135.7203) -> (150.2998, 135.6443) construction
  line L5725 (150.2998, 135.6443) -> (150.1623, 135.5673) construction